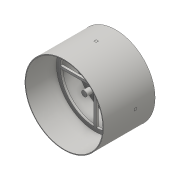
# Autodesk Inventor part: control surfaces
Saved by Autodesk Inventor 2016 (Build 200138000, 138)
## iProperties
Created: 2016-06-08
Part Number: control surfaces
Material: Generic
Document SubType Name: Modeling
Designer: s_sud
Density: 1 g/cm^3
Appearance: Default
Author: s_sud
Autodesk Inventor part; units mm, degrees
ref_plane "YZ Plane" through (0, 0, 0) normal (1, 0, 0) x (0, 1, 0)
ref_plane "XZ Plane" through (0, 0, 0) normal (0, 1, 0) x (-1, 0, 0)
ref_plane "XY Plane" through (0, 0, 0) normal (0, 0, 1) x (1, 0, 0)
sketch "Sketch1" plane through (0, 0, 0) normal (0, 1, 0) x (-1, 0, 0)
  circle A0 centre (0, 0) radius 45
  circle A1 centre (0, 0) radius 51
  dimension "d0" = 90
  dimension "d1" = 102
  constraints: 2 centre point, 2 coincident
  measures "d0" diameter of A0
  measures "d1" diameter of A1
extrude "Extrusion1" add sketch "Sketch1" along normal blind 3
sketch "Sketch2" plane through (0, 0, 0) normal (0, -1, 0) x (1, 0, 0)
  circle A0 centre (0, 0) radius 50
  circle A1 centre (0, 0) radius 51
  dimension "d4" = 100
  dimension "d5" = 102
  constraints: 2 centre point, 2 coincident
  measures "d4" diameter of A0
  measures "d5" diameter of A1
extrude "Extrusion2" add sketch "Sketch2" along normal blind 40 and the other way blind 25
sketch "Sketch3" plane through (0, 3, 0) normal (0, 1, 0) x (1, 0, 0)
  line L0 (1.5, 51) -> (-1.5, 51)
  line L1 (-1.5, 51) -> (-1.5, -51)
  line L2 (-1.5, -51) -> (1.5, -51)
  line L3 (1.5, -51) -> (1.5, 51)
  line L4 (1.5, 51) -> (-1.5, -51) construction
  line L5 (-1.5, 51) -> (1.5, -51) construction
  line L6 (-51, 1.5) -> (51, 1.5)
  line L7 (51, 1.5) -> (51, -1.5)
  line L8 (51, -1.5) -> (-51, -1.5)
  line L9 (-51, -1.5) -> (-51, 1.5)
  line L10 (-51, 1.5) -> (51, -1.5) construction
  line L11 (51, 1.5) -> (-51, -1.5) construction
  point P0 (0, 0)
  dimension "d8" = 3
  dimension "d9" = 102
  dimension "d10" = 102
  dimension "d11" = 3
  constraints: 24 end point, 4 midpoint, 4 parallel, 2 horizontal, 2 perpendicular
  measures "d8" distance of L2.end L1.end
  measures "d9" distance of L0.end L1.end
  measures "d10" distance of L7.end L8.end
  measures "d11" distance of L8.end L6.start
extrude "Extrusion3" add sketch "Sketch3" against normal blind 3
sketch "Sketch4" plane through (0, 25, 0) normal (0, 1, 0) x (1, 0, 0)
  circle A0 centre (0, 0) radius 51
  circle A1 centre (0, 0) radius 40.5
  dimension "d59" = 81
  dimension "d60" = 102
  constraints: 2 centre point, 2 coincident
  measures "d59" diameter of A1
  measures "d60" diameter of A0
extrude "Extrusion4" add sketch "Sketch4" along normal blind 2
sketch "Sketch5" plane through (0, 27, 0) normal (0, 1, 0) x (1, 0, 0)
  line L0 (0, 0) -> (0, -9.8522)
  line L1 (-1.5, -44.975) -> (-1.5, -1.5) projected
  line L2 (0, 0) -> (7.9084, -7.9084)
  circle A0 centre (31, -31.4363) radius 2.5
  circle A1 centre (31.4363, 31) radius 2.5
  circle A2 centre (-31, 31.4363) radius 2.5
  circle A3 centre (-31.4363, -31) radius 2.5
  circle A4 centre (31, -31.4363) radius 3.5
  circle A5 centre (31.4363, 31) radius 3.5
  circle A6 centre (-31, 31.4363) radius 3.5
  circle A7 centre (-31.4363, -31) radius 3.5
  dimension "d18" = 45
  dimension "d19" = 5
  dimension "d20" = 31
  dimension "d23" = 360
  dimension "d25" = 7
  dimension "d28" = 360
  constraints: 8 centre point, 4 end point, 1 coincident, 1 parallel, 18 other
  measures "d18" angle of L0 L2
  measures "d19" diameter of A0
  measures "d20" horizontal distance of A0.centre L0.start
  measures "d25" diameter of A4
extrude "Extrusion5" add sketch "Sketch5" against normal blind 10 contours A0 | A4
pattern_circular "Circular Pattern1" count 4 over 360 about axis through (0, -10, 0) along (0, 1, 0) of "Extrusion5"
sketch "Sketch7" plane through (0, 27, 0) normal (0, 1, 0) x (1, 0, 0)
  line L0 (0, 0) -> (0, -9.8522)
  line L1 (-1.5, -38.4708) -> (-1.5, -1.5)
  line L2 (0, 0) -> (7.9084, -7.9084)
  circle A0 centre (31, -31.4363) radius 2.5
  circle A1 centre (31.4363, 31) radius 2.5
  circle A2 centre (-31, 31.4363) radius 2.5
  circle A3 centre (-31.4363, -31) radius 2.5
  circle A4 centre (31, -31.4363) radius 3.5
  circle A5 centre (31.4363, 31) radius 3.5
  circle A6 centre (-31, 31.4363) radius 3.5
  circle A7 centre (-31.4363, -31) radius 3.5
  dimension "d51" = 45
  dimension "d52" = 5
  dimension "d53" = 31
  dimension "d54" = 360
  dimension "d55" = 7
  dimension "d56" = 360
  constraints: 8 centre point, 6 end point, 1 coincident, 1 parallel, 18 other
  measures "d51" angle of L0 L2
  measures "d52" diameter of A0
  measures "d53" horizontal distance of A0.centre L0.start
  measures "d55" diameter of A4
extrude "Extrusion7" cut sketch "Sketch7" against normal blind 8 contours A0 | A1 | A2 | A3
body "Solid1"
